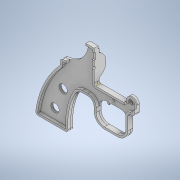
# Autodesk Inventor part: Telo_Levo_1
Saved by Autodesk Inventor 2021 (Build 250183000, 183)
## iProperties
Created: 2022-03-04
Part Number: Telo_Levo_1
Material: Generic
Document SubType Name: Modeling
Designer: Carlos Montoya
Density: 1 g/cm^3
Appearance: Default
Author: Carlos Montoya
Autodesk Inventor part; units mm, degrees
ref_plane "YZ Plane" through (0, 0, 0) normal (1, 0, 0) x (0, 1, 0)
ref_plane "XZ Plane" through (0, 0, 0) normal (0, 1, 0) x (-1, 0, 0)
sketch "Sketch1" plane through (0, 0, 0) normal (0, 0, 1) x (1, 0, 0)
  arc A0 (10.5, -12.5) -> (0.5, -22.5) centre (10.5, -22.5) ccw
  line L0 (0.5, -27.5) -> (0.5, -22.5)
  arc A1 (0.5, -27.5) -> (10.5, -37.5) centre (10.5, -27.5) ccw
  line L1 (26.5, -37.5) -> (10.5, -37.5)
  arc A2 (26.5, -37.5) -> (36.5, -27.5) centre (26.5, -27.5) ccw
  line L2 (36.5, -22.5) -> (36.5, -27.5)
  arc A3 (36.5, -22.5) -> (26.5, -12.5) centre (26.5, -22.5) ccw
  line L3 (10.5, -12.5) -> (26.5, -12.5)
  line L4 (39, -12) -> (39, -27.5)
  arc A4 (26.5, -40) -> (39, -27.5) centre (26.5, -27.5) ccw
  line L5 (26.5, -40) -> (10.5, -40)
  arc A5 (-2, -27.5) -> (10.5, -40) centre (10.5, -27.5) ccw
  line L6 (-2, -27.5) -> (-2, -22.5)
  arc A6 (-2, -22.5) -> (-9.5, -15) centre (-9.5, -22.5) ccw
  line L7 (-9.5, -15) -> (-16.1314, -15)
  arc A7 (-16.1314, -15) -> (-24.9209, -20.2308) centre (-16.1314, -25) ccw
  arc A8 (-24.9209, -20.2308) -> (-33.6974, -62.7308) centre (41, -56) ccw
  arc A9 (-36.6853, -66) -> (-33.6974, -62.7308) centre (-36.6853, -63) ccw
  line L8 (-36.6853, -66) -> (-69.991, -66)
  arc A10 (-43.7881, -0.3085) -> (-72.964, -62.5982) centre (41, -78) ccw
  arc A11 (-72.964, -62.5982) -> (-69.991, -66) centre (-69.991, -63) ccw
  line L9 (-43, 5.1326) -> (-43, 1.7183)
  arc A12 (-43.7881, -0.3085) -> (-43, 1.7183) centre (-46, 1.7183) ccw
  arc A13 (-40.2647, 8.1209) -> (-43, 5.1326) centre (-40, 5.1326) ccw
  arc A14 (-40.2647, 8.1209) -> (-12.1982, 35.5) centre (-43, 39) ccw
  line L10 (-12.1982, 35.5) -> (-2, 35.5)
  arc A15 (-2, 2) -> (0, 0) centre (0, 2) ccw
  line L11 (0, 0) -> (34, 0)
  arc A16 (34, 0) -> (35, 1) centre (34, 1) ccw
  arc A17 (47, 2) -> (35, 2) centre (41, 2) ccw
  line L12 (35, 1) -> (35, 2)
  arc A18 (44, -9) -> (47, -6) centre (44, -6) ccw
  line L13 (44, -9) -> (42, -9)
  arc A19 (42, -9) -> (39, -12) centre (42, -12) ccw
  circle A20 centre (-43, -26) radius 5
  circle A21 centre (-53, -51) radius 5
  circle A22 centre (41, 2) radius 1.75
  line L14 (-2, 2) -> (-2, 35.5)
  line L15 (47, 2) -> (47, -6)
  point P0 (0, 0)
  dimension "d2" = 10.1982
  dimension "d3" = 33.5
  dimension "d4" = 31
  dimension "d5" = 3
  dimension "d6" = 3.4144
  dimension "d7" = 3
  dimension "d8" = 115
  dimension "d9" = 3
  dimension "d10" = 3
  dimension "d11" = 33.3057
  dimension "d12" = 10
  dimension "d13" = 10
  dimension "d14" = 75
  dimension "d15" = 10
  dimension "d16" = 6.6314
  dimension "d17" = 7.5
  dimension "d18" = 5
  dimension "d19" = 12.5
  dimension "d20" = 16
  dimension "d21" = 12.5
  dimension "d22" = 15.5
  dimension "d23" = 3
  dimension "d25" = 3
  dimension "d26" = 8
  dimension "d27" = 6
  dimension "d28" = 3.5
  dimension "d29" = 1
  dimension "d30" = 34
  dimension "d33" = 1
  dimension "d35" = 1
  dimension "d36" = 2
  dimension "d37" = 2
  dimension "d38" = 2
  dimension "d39" = 28.0665
  dimension "d40" = 27.3791
  dimension "d41" = 2.9883
  dimension "d42" = 2.7353
  dimension "d43" = 0.7881
  dimension "d44" = 2.0267
  dimension "d45" = 12
  dimension "d46" = 2
  dimension "d47" = 6
  dimension "d48" = 3
  dimension "d49" = 3
  dimension "d52" = 3
  dimension "d53" = 3
  dimension "d57" = 3
  dimension "d58" = 3
  dimension "d59" = 2
  dimension "d60" = 5
  dimension "d61" = 27.5
  dimension "d62" = 12.5
  dimension "d63" = 12.5
  dimension "d64" = 12.5
  dimension "d65" = 12.5
  dimension "d66" = 36
  dimension "d67" = 5
  dimension "d68" = 5
  dimension "d69" = 16
  dimension "d70" = 16
  dimension "d71" = 10
  dimension "d72" = 10
  dimension "d73" = 22.5
  dimension "d74" = 25
  constraints: 40 point on circle, 32 end point, 23 centre point, 4 vertical, 2 coincident, 2 horizontal, 1 horizontal alignment, 1 perpendicular
  measures "d2" distance of L10.start L10.end
  measures "d3" distance of L14.start L10.end
  measures "d4" radius of A14
  measures "d5" radius of A13
  measures "d6" distance of L9.start L9.end
  measures "d7" radius of A12
  measures "d8" radius of A10
  measures "d9" radius of A11
  measures "d10" radius of A9
  measures "d11" distance of L8.start L8.end
  measures "d12" diameter of A21
  measures "d13" diameter of A20
  measures "d14" radius of A8
  measures "d15" radius of A7
  measures "d16" distance of L7.start L7.end
  measures "d17" radius of A6
  measures "d18" distance of L6.start L6.end
  measures "d19" radius of A5
  measures "d20" distance of L5.start L5.end
  measures "d21" radius of A4
  measures "d22" distance of L4.start L4.end
  measures "d23" radius of A19
  measures "d25" radius of A18
  measures "d26" distance of L15.start L15.end
  measures "d27" radius of A17
  measures "d28" diameter of A22
  measures "d29" radius of A16
  measures "d30" distance of L11.start L11.end
  measures "d33" horizontal distance of L12.start L11.end
  measures "d35" horizontal distance of L11.end L12.start
  measures "d36" horizontal distance of L11.start L14.start
  measures "d37" horizontal distance of L11.start L14.start
  measures "d38" radius of A15
  measures "d39" horizontal distance of A13.start L10.start
  measures "d40" vertical distance of A13.start L10.start
  measures "d41" vertical distance of L9.start A13.start
  measures "d42" horizontal distance of A13.start L9.start
  measures "d43" horizontal distance of A12.start L9.end
  measures "d44" vertical distance of A12.start L9.end
  measures "d45" distance of L15.start L12.end
  measures "d46" distance from line of L11 A17.centre
  measures "d47" horizontal distance of L12.start A17.centre
  measures "d48" distance of L15.end A18.centre
  measures "d49" distance of L13.start A18.centre
  measures "d52" horizontal distance of L15.end L13.start
  measures "d53" horizontal distance of L13.start L15.end
  measures "d57" distance of A19.centre L13.end
  measures "d58" distance of L4.start A19.centre
  measures "d59" distance of L13.start L13.end
  measures "d60" horizontal distance of L13.start L4.start
  measures "d61" vertical distance of L4.end point (0, 0)
  measures "d62" distance of L4.end A2.centre
  measures "d63" distance of L5.start A2.centre
  measures "d64" horizontal distance of L5.start L4.end
  measures "d65" horizontal distance of L5.start L4.end
  measures "d66" distance between parallel lines of L2 L0
  measures "d67" distance of L0.start L0.end
  measures "d68" distance of L2.end L2.start
  measures "d69" distance of L3.start L3.end
  measures "d70" distance of L1.start L1.end
  measures "d71" radius of A0
  measures "d72" radius of A3
  measures "d73" vertical distance of A0.centre L11.start
  measures "d74" distance of L1.end L3.start
extrude "Extrusion1" add sketch "Sketch1" along normal blind 2.5
sketch "Sketch2" plane through (0, 0, 2.5) normal (0, 0, 1) x (1, 0, 0)
  arc A0 (-41.9449, -1.9974) -> (-70.4865, -62.933) centre (41, -78) ccw
  arc A1 (-43.7881, -0.3085) -> (-72.964, -62.5982) centre (41, -78) ccw
  line L0 (-43, 5.1326) -> (-43, 1.7183)
  arc A2 (-43.7881, -0.3085) -> (-43, 1.7183) centre (-46, 1.7183) ccw
  arc A3 (-40.2647, 8.1209) -> (-43, 5.1326) centre (-40, 5.1326) ccw
  arc A4 (-40.2647, 8.1209) -> (-35, 9.05) centre (-43, 39) ccw
  arc A5 (-40.0441, 5.6307) -> (-35, 6.4692) centre (-43, 39) ccw
  line L1 (-40.5, 5.1326) -> (-40.5, 1.7183)
  arc A6 (-40.0441, 5.6307) -> (-40.5, 5.1326) centre (-40, 5.1326) ccw
  line L2 (-35, 9.05) -> (-35, 6.4692)
  arc A7 (-41.9449, -1.9974) -> (-40.5, 1.7183) centre (-46, 1.7183) ccw
  arc A8 (-72.964, -62.5982) -> (-69.991, -66) centre (-69.991, -63) ccw
  arc A9 (-70.4865, -62.933) -> (-69.991, -63.5) centre (-69.991, -63) ccw
  line L3 (-36.6853, -63.5) -> (-69.991, -63.5)
  arc A10 (-36.6853, -63.5) -> (-36.1873, -62.9551) centre (-36.6853, -63) ccw
  arc A11 (-27.1182, -19.0385) -> (-36.1873, -62.9551) centre (41, -56) ccw
  line L4 (-36.6853, -66) -> (-69.991, -66)
  arc A12 (-36.6853, -66) -> (-33.6974, -62.7308) centre (-36.6853, -63) ccw
  arc A13 (-24.9209, -20.2308) -> (-33.6974, -62.7308) centre (41, -56) ccw
  arc A14 (-16.1314, -12.5) -> (-27.1182, -19.0385) centre (-16.1314, -25) ccw
  arc A15 (-16.1314, -15) -> (-24.9209, -20.2308) centre (-16.1314, -25) ccw
  line L5 (-9.5, -15) -> (-16.1314, -15)
  line L6 (-9.5, -12.5) -> (-16.1314, -12.5)
  arc A16 (0.5, -22.5) -> (-9.5, -12.5) centre (-9.5, -22.5) ccw
  arc A17 (-2, -22.5) -> (-9.5, -15) centre (-9.5, -22.5) ccw
  line L7 (-2, -27.5) -> (-2, -22.5)
  line L8 (0.5, -27.5) -> (0.5, -22.5)
  arc A18 (-2, -27.5) -> (10.5, -40) centre (10.5, -27.5) ccw
  arc A19 (0.5, -27.5) -> (10.5, -37.5) centre (10.5, -27.5) ccw
  line L9 (26.5, -37.5) -> (10.5, -37.5)
  line L10 (26.5, -40) -> (10.5, -40)
  arc A20 (26.5, -40) -> (39, -27.5) centre (26.5, -27.5) ccw
  arc A21 (26.5, -37.5) -> (36.5, -27.5) centre (26.5, -27.5) ccw
  line L11 (36.5, -12) -> (36.5, -27.5)
  line L12 (39, -12) -> (39, -27.5)
  arc A22 (42, -6.5) -> (36.5, -12) centre (42, -12) ccw
  arc A23 (42, -9) -> (39, -12) centre (42, -12) ccw
  arc A24 (44, -9) -> (47, -6) centre (44, -6) ccw
  line L13 (44.5, -4.0622) -> (44.5, -6)
  line L14 (44, -9) -> (42, -9)
  line L15 (44, -6.5) -> (42, -6.5)
  arc A25 (44, -6.5) -> (44.5, -6) centre (44, -6) ccw
  line L16 (47, -1.6056) -> (47, -6)
  arc A26 (44.5, -4.0622) -> (47, -1.6056) centre (41, 2) ccw
  line L17 (0, 0) -> (34, 0)
  line L18 (0, -2.5) -> (34, -2.5)
  arc A27 (34.28, 0.04) -> (35.4044, -2.2059) centre (41, 2) ccw
  arc A28 (34, -2.5) -> (35.4044, -2.2059) centre (34, 1) ccw
  arc A29 (34, 0) -> (34.28, 0.04) centre (34, 1) ccw
  arc A30 (-4.5, 2) -> (0, -2.5) centre (0, 2) ccw
  arc A31 (-2, 2) -> (0, 0) centre (0, 2) ccw
  line L19 (-4.5, 16.5) -> (-4.5, 2)
  line L20 (-2, 16.5) -> (-2, 2)
  line L21 (-4.5, 16.5) -> (-2, 16.5)
  line L22 (-4.5, 19.5) -> (-2, 19.5)
  line L23 (-4.5, 26) -> (-4.5, 19.5)
  line L24 (-2, 26) -> (-2, 19.5)
  line L25 (-4.5, 26) -> (-2, 26)
  line L26 (-4.5, 34) -> (-2, 34)
  line L27 (-4.5, 36.5) -> (-4.5, 34)
  line L28 (-2, 39) -> (-2, 34)
  line L29 (-2, 39) -> (-12, 39)
  arc A32 (-12.101, 36.5) -> (-12, 39) centre (-43, 39) ccw
  line L30 (-4.5, 36.5) -> (-12.101, 36.5)
  circle A33 centre (18, -8) radius 1.5
  point P0 (0, 0)
  constraints: 66 point on circle, 62 end point, 34 centre point
extrude "Extrusion2" add sketch "Sketch2" along normal blind 3.5
sketch "Sketch3" plane through (0, 0, 2.5) normal (0, 0, 1) x (1, 0, 0)
  arc A0 (35.4044, -2.2059) -> (37.5, 1) centre (34, 1) ccw
  arc A1 (34.28, 0.04) -> (35, 1) centre (34, 1) ccw
  arc A2 (34.28, 0.04) -> (35.4044, -2.2059) centre (41, 2) ccw
  line L0 (35, 2) -> (35, 1)
  arc A3 (47, 2) -> (35, 2) centre (41, 2) ccw
  line L1 (37.5, 1) -> (37.5, 2)
  arc A4 (44.5, 2) -> (37.5, 2) centre (41, 2) ccw
  line L2 (44.5, 2) -> (44.5, -4.0622)
  line L3 (47, -1.6056) -> (47, 2)
  arc A5 (44.5, -4.0622) -> (47, -1.6056) centre (41, 2) ccw
  circle A6 centre (41, 2) radius 1.75
  circle A7 centre (41, 2) radius 2.5
  point P0 (0, 0)
  constraints: 12 point on circle, 8 centre point, 8 end point
extrude "Extrusion3" add sketch "Sketch3" along normal blind 1
sketch "Sketch4" plane through (18, -8, 6) normal (0, 0, 1) x (1, 0, 0)
  circle A0 centre (0, 0) radius 1.5
  point P0 (-18, 8)
  constraints: 1 centre point
extrude "Extrusion4" add sketch "Sketch4" along normal blind 2.5
sketch "Sketch5" plane through (0, 0, 2.5) normal (0, 0, -1) x (-1, 0, 0)
  point P0 (0, 0)
sketch "Sketch6" plane through (0, 0, 2.5) normal (0, 0, 1) x (1, 0, 0)
  line L0 (-2, 39) -> (-2, 35.5)
  line L1 (-12, 39) -> (-2, 39)
  line L2 (-12.1982, 35.5) -> (-2, 35.5)
  arc A0 (-12.1982, 35.5) -> (-12, 39) centre (-43, 39) ccw
  point P0 (0, 0)
  constraints: 6 end point, 2 point on circle, 1 centre point
extrude "Extrusion5" add sketch "Sketch6" against normal blind 1.5
sketch "Sketch7" plane through (0, 0, 2.5) normal (0, 0, 1) x (1, 0, 0)
  line L0 (-2, 34) -> (-4.5, 34) projected
  line L1 (-4.5, 26) -> (-2, 26) projected
  line L2 (-4.5, 34) -> (-2, 34)
  line L3 (-2, 34) -> (-2, 26)
  line L4 (-2, 26) -> (-4.5, 26)
  line L5 (-4.5, 26) -> (-4.5, 34)
  point P0 (0, 0)
  constraints: 8 end point, 2 parallel, 1 horizontal, 1 perpendicular
extrude "Extrusion6" add sketch "Sketch7" along normal blind 2
sketch "Sketch8" plane through (0, 0, 2.5) normal (0, 0, 1) x (1, 0, 0)
  line L0 (-2, 19.5) -> (-4.5, 19.5) projected
  line L1 (-4.5, 19.5) -> (-2, 19.5)
  line L2 (-2, 19.5) -> (-2, 16.5)
  line L3 (-2, 16.5) -> (-4.5, 16.5)
  line L4 (-4.5, 16.5) -> (-4.5, 19.5)
  point P0 (0, 0)
  constraints: 8 end point, 2 parallel, 1 horizontal, 1 perpendicular
extrude "Extrusion7" add sketch "Sketch8" along normal blind 3.5
sketch "Sketch9" plane through (-4.5, 2, 2.5) normal (-1, 0, 0) x (0, 0, 1)
  arc A0 (3.5, 17.5) -> (3.5, 14.5) centre (3.5, 16) ccw
  line L0 (3.5, 24) -> (3.5, 17.5)
  line L1 (3.5, 14.5) -> (3.5, 0)
  line L2 (2, 24) -> (2, 7.05)
  line L3 (0, 7.05) -> (3.5, 7.05) projected
  line L4 (3.5, 14.5) -> (3.5, 17.5) projected
  line L5 (3.5, 0) -> (3.5, 14.5) projected
  line L6 (3.5, 17.5) -> (3.5, 14.5)
  point P0 (-2.5, -2)
  constraints: 8 end point, 2 point on circle, 1 centre point, 1 collinear, 1 point on line, 1 vertical
extrude "Extrusion8" cut sketch "Sketch9" against normal blind 3.5 contours L4 A0
fillet "Fillet1" radius 0.4125 1 edges at (16.5, -8, 8.5)
chamfer "Chamfer2" distance 2 angle 45 1 edges at (39.25, 2, 0)
ref_plane "Work Plane1" through (-2, 18, 4.5) normal (0, 1, 0) x (1, 0, 0)
sketch "Sketch14" plane through (-2, 18, 4.5) normal (0, 1, 0) x (1, 0, 0)
  arc A0 (0.6654, -14.5) -> (6.9706, -6) centre (-10, 0) ccw
  line L0 (0.6654, -14.5) -> (0.6654, -6)
  line L1 (0.6654, -6) -> (6.9706, -6)
  line L2 (0, 4.5) -> (-6.305, 4.5)
  line L3 (0, 3.5) -> (0, -1.5) projected
  line L4 (0, 4.5) -> (0, 2) projected
  line L5 (0, 4.5) -> (-0.665, 4.5)
  line L6 (0, 4.5) -> (-7.5, 4.5) projected
  line L7 (-0.665, 4.5) -> (-0.665, 13)
  line L8 (-0.665, 4.5) -> (-6.97, 4.5)
  arc A1 (-0.665, 13) -> (-6.97, 4.5) centre (10.0006, -1.4998) ccw
  line L9 (10.0006, -1.4998) -> (10.0006, 12.3282)
  line L10 (-0.665, 13) -> (10.0006, 13)
  line L11 (10.0006, 13) -> (10.0006, 12.3282)
  line L12 (-0.665, 4.5) -> (10.0006, 4.5)
  line L13 (0, 4.5) -> (12.5, 4.5) projected
  line L14 (0, 4.5) -> (0, 13)
  dimension "d110" = 6.3052
  dimension "d111" = 90
  dimension "d115" = 0.665
  dimension "d116" = 8.5
  dimension "d117" = 6.305
  dimension "d118" = 18
  constraints: 22 end point, 5 point on line, 4 point on circle, 3 perpendicular, 2 centre point, 2 horizontal, 1 vertical, 4 other
  measures "d110" distance of L1.end L0.end
  measures "d111" angle of L1 L0
  measures "d115" distance of L2.start L5.end
  measures "d116" distance of L5.end L7.end
  measures "d117" distance of L5.end L8.end
  measures "d118" radius of A1
revolve "Revolution1" add sketch "Sketch14" angle 180 mid plane about axis through (8.0006, 18, 5.9998) along (0, 0, -1) contours L14 L10 L11 L9 L12 | L2 L7 L10 L14 | L2 L6 A1 L7
sketch "Sketch15" plane through (-2, 18, 4.5) normal (0, 1, 0) x (1, 0, 0)
  arc A0 (0.6654, -14.5) -> (6.9706, -6) centre (-10, 0) ccw
  line L0 (0.6654, -14.5) -> (0.6654, -6)
  line L1 (0.6654, -6) -> (6.9706, -6)
  line L2 (0, 4.5) -> (-6.305, 4.5)
  line L3 (0, 3.5) -> (0, -1.5)
  line L4 (0, 4.5) -> (0, 2)
  line L5 (0, 4.5) -> (-0.665, 4.5)
  line L6 (0, 4.5) -> (-7.5, 4.5)
  line L7 (-0.665, 4.5) -> (-0.665, 13)
  line L8 (-0.665, 4.5) -> (-6.97, 4.5)
  arc A1 (-0.665, 13) -> (-6.97, 4.5) centre (10.0006, -1.4998) ccw
  line L9 (10.0006, -1.4998) -> (10.0006, 12.3282)
  line L10 (-0.665, 13) -> (10.0006, 13)
  line L11 (10.0006, 13) -> (10.0006, 12.3282)
  line L12 (-0.665, 4.5) -> (10.0006, 4.5)
  line L13 (0, 4.5) -> (12.5, 4.5)
  line L14 (0, 4.5) -> (0, 13)
  line L15 (-0.665, 13) -> (-0.665, 4.5)
  line L16 (-7.5, -1.5) -> (2.5, -1.5) projected
  line L17 (0, 13) -> (0, 4.5)
  line L18 (0, 4.5) -> (-0.665, 4.5)
  line L19 (-0.665, 4.5) -> (14.1924, 4.5)
  line L20 (14.1924, 4.5) -> (14.1924, 14.2692)
  line L21 (14.1924, 14.2692) -> (-0.665, 14.2692)
  line L22 (-0.665, 14.2692) -> (-0.665, 4.5)
  point P0 (2, 4.5)
  point P1 (0, 4.5)
  point P2 (-0.665, 13)
  point P3 (-0.665, 4.5)
  point P4 (0, 4.5)
  dimension "d120" = 6.3052
  dimension "d121" = 90
  dimension "d122" = 0.665
  dimension "d123" = 8.5
  dimension "d124" = 6.305
  dimension "d125" = 18
  constraints: 44 end point, 7 perpendicular, 5 point on line, 4 point on circle, 3 horizontal, 2 centre point, 2 parallel, 1 vertical, 4 other
  measures "d120" distance of L1.end L0.end
  measures "d121" angle of L1 L0
  measures "d122" distance of L2.start L5.end
  measures "d123" distance of L5.end L7.end
  measures "d124" distance of L5.end L8.end
  measures "d125" radius of A1
extrude "Extrusion9" cut sketch "Sketch15" against normal mid plane 50 contours L14 L10 L11 L9 L12 | L2 L7 L10 L14 | L9 L11 L10 L22 L21 L20 L19 L13
sketch "Sketch17" plane through (-2.665, 18, 5.9998) normal (1, 0, 0) x (0, 0, -1)
  arc A0 (5.9998, -13.2003) -> (5.9998, 13.2003) centre (0, 0) ccw projected
  line L0 (5.9998, 13.2003) -> (5.9998, -13.2003) projected
  point P0 (5.9998, -18)
extrude "Extrusion10" add sketch "Sketch17" along normal blind 0.665
body "Solid1"
